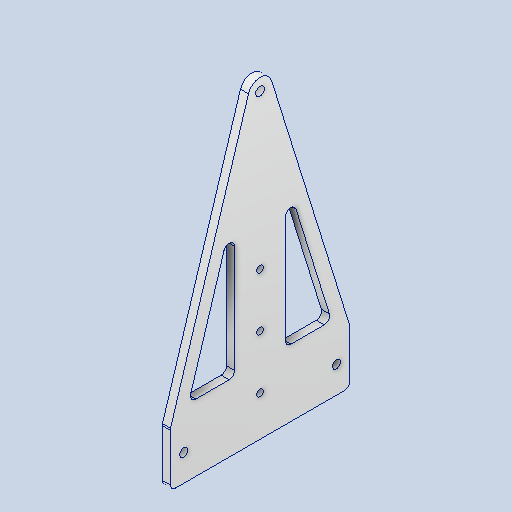
# Autodesk Inventor part: odom_v1_Plate_5
Saved by Autodesk Inventor 2025.2 (Build 292293000, 293)
## iProperties
Created: 2025-04-01
Part Number: odom_v1_Plate_5
Material: アルミニウム 6061
Document SubType Name: Modeling
Designer: haruy
Density: 2.7 g/cm^3
Appearance: アルミニウム - フラット
Author: haruy
Autodesk Inventor part; units mm, degrees
ref_plane "YZ Plane" through (0, 0, 0) normal (1, 0, 0) x (0, 1, 0)
ref_plane "XZ Plane" through (0, 0, 0) normal (0, 1, 0) x (-1, 0, 0)
ref_plane "XY Plane" through (0, 0, 0) normal (0, 0, 1) x (1, 0, 0)
derived "odom_v1_Sketch_Base.ipt"
sketch "スケッチ1" plane through (300, 0, 0) normal (1, 0, 0) x (0, 1, 0)
  line L0 (0, 0) -> (20, 0)
  line L1 (20, 0) -> (20, -192.6893)
  line L2 (20, -192.6893) -> (0, -192.6893)
  line L3 (0, -192.6893) -> (0, 0)
  line L4 (-77, 0) -> (-77, -265.1297)
  circle A0 centre (7.5, -57.9764) radius 1.6
  circle A1 centre (7.5, -93.4764) radius 1.6
  line L5 (-20, -52.2264) -> (-66, -52.2264)
  line L6 (-66, -52.2264) -> (-66, -57.2264)
  line L7 (-66, -57.2264) -> (-20, -57.2264)
  line L8 (-20, -57.2264) -> (-20, -52.2264)
  line L9 (-20, -94.2264) -> (-66, -94.2264)
  line L10 (-66, -94.2264) -> (-66, -99.2264)
  line L11 (-66, -99.2264) -> (-20, -99.2264)
  line L12 (-20, -99.2264) -> (-20, -94.2264)
  line L13 (-19.371, -66.7264) -> (-77, -66.7264)
  line L14 (-77, -66.7264) -> (-77, -84.7264)
  line L15 (-77, -84.7264) -> (-19.371, -84.7264)
  line L16 (-19.371, -84.7264) -> (-19.371, -66.7264)
  line L17 (-41.1855, -57.2264) -> (-55.1855, -57.2264)
  line L18 (-55.1855, -57.2264) -> (-55.1855, -58.0264)
  line L19 (-55.1855, -58.0264) -> (-41.1855, -58.0264)
  line L20 (-41.1855, -58.0264) -> (-41.1855, -57.2264)
  line L21 (-48.1855, -66.7264) -> (-48.1855, -84.7264)
  line L22 (-55.1855, -94.2264) -> (-41.1855, -94.2264)
  line L23 (-41.1855, -94.2264) -> (-41.1855, -93.4264)
  line L24 (-41.1855, -93.4264) -> (-55.1855, -93.4264)
  line L25 (-55.1855, -93.4264) -> (-55.1855, -94.2264)
  circle A2 centre (48, -75.7264) radius 1.65
  circle A3 centre (-17, -75.7264) radius 2
  line L26 (48, -75.7264) -> (-17, -75.7264)
  line L27 (33.5, -67.2264) -> (-12, -67.2264)
  line L28 (-12, -67.2264) -> (-12, -84.2264)
  line L29 (-12, -84.2264) -> (33.5, -84.2264)
  line L30 (33.5, -84.2264) -> (33.5, -67.2264)
  line L31 (-12, -73.7264) -> (-20, -73.7264)
  line L32 (-20, -73.7264) -> (-20, -77.7264)
  line L33 (-20, -77.7264) -> (-12, -77.7264)
  line L34 (-12, -77.7264) -> (-12, -73.7264)
  line L35 (-2, -71.2264) -> (-57, -71.2264)
  line L36 (-57, -71.2264) -> (-57, -80.2264)
  line L37 (-57, -80.2264) -> (-2, -80.2264)
  line L38 (-2, -80.2264) -> (-2, -71.2264)
  circle A4 centre (-9.5, -75.7264) radius 1.25
  circle A5 centre (-29.5, -75.7264) radius 1.25
  circle A6 centre (-49.5, -75.7264) radius 1.25
  line L39 (-52, -65.7264) -> (-22, -65.7264)
  line L40 (-22, -65.7264) -> (-22, -85.7264)
  line L41 (-22, -85.7264) -> (-52, -85.7264)
  line L42 (-52, -85.7264) -> (-52, -65.7264)
  line L43 (-43, -52.2264) -> (-43, -57.2264)
  circle A7 centre (-33, -54.7264) radius 1.5
  line L44 (-29.5, -75.7264) -> (-49.5, -75.7264)
  circle A8 centre (-53, -54.7264) radius 1.5
  circle A9 centre (-53, -96.7264) radius 1.5
  circle A10 centre (-33, -96.7264) radius 1.5
  line L45 (-44.5, -42.2264) -> (-64.5, -42.2264)
  line L46 (-64.5, -42.2264) -> (-64.5, -109.2264)
  line L47 (-64.5, -109.2264) -> (-44.5, -109.2264)
  line L48 (-44.5, -109.2264) -> (-44.5, -42.2264)
  circle A11 centre (-54.5, -47.2264) radius 1.5
  circle A12 centre (-54.5, -104.2264) radius 1.5
  circle A13 centre (48, -75.7264) radius 4.5
  line L49 (48, -71.2264) -> (-2, -71.2264)
  line L50 (-2, -80.2264) -> (48, -80.2264)
  line L51 (-44.5, -42.2264) -> (49.3372, -71.4297)
  line L52 (-39.5, -37.2264) -> (-69.5, -37.2264)
  line L53 (-69.5, -37.2264) -> (-69.5, -114.2264)
  line L54 (-69.5, -114.2264) -> (-39.5, -114.2264)
  line L55 (-39.5, -114.2264) -> (-39.5, -37.2264)
  line L56 (-45.9858, -47.0006) -> (47.8514, -76.2038)
  line L57 (48, -66.2264) -> (-2, -66.2264)
  line L58 (-62, -66.2264) -> (3, -66.2264)
  line L59 (3, -66.2264) -> (3, -85.2264)
  line L60 (3, -85.2264) -> (-62, -85.2264)
  line L61 (-62, -85.2264) -> (-62, -66.2264)
  line L62 (33.5, -84.2264) -> (-12, -84.2264)
  line L63 (-44.5, -109.2264) -> (49.3372, -80.0232)
  line L64 (-39.5, -37.2264) -> (-39.5, -114.2264)
  line L65 (-45.9858, -104.4523) -> (47.8514, -75.249)
  line L66 (48, -85.2264) -> (-2, -85.2264)
  line L67 (-62, -85.2264) -> (3, -85.2264)
  point P0 (-44.5, -71.2264)
  point P1 (-44.5, -80.2264)
  point P2 (-39.5, -85.2264)
  point P3 (15.7916, -85.2264)
  point P4 (-20, -96.3652)
  point P5 (-29.1938, -99.2264)
  point P6 (-39.5, -102.4338)
  point P7 (49.3372, -80.0232)
  point P8 (-39.5, -49.019)
  point P9 (15.7916, -66.2264)
  point P10 (-2, -66.2264)
  point P11 (-39.5, -66.2264)
  point P12 (8.853, -58.8305)
  point P13 (5.9013, -57.9119)
  dimension "d1" = 20
  dimension "d2" = 12.5
  dimension "d3" = 3
  dimension "d4" = 3
  dimension "d5" = 10
  dimension "d7" = 10
  dimension "d10" = 5
  dimension "d11" = 5
  dimension "d12" = 5
  dimension "d13" = 5
  dimension "d14" = 9
  dimension "d17" = 5
  dimension "d18" = 5
  dimension "d19" = 5
  dimension "d20" = 5
  measures "d1" distance of L47.end L46.end
  measures "d2" distance between parallel lines of L4 L46
  measures "d3" diameter of A11
  measures "d4" diameter of A12
  measures "d5" distance from line of A11.centre L46
  measures "d7" distance from line of A12.centre L46
  measures "d10" distance from line of A11.centre L45
  measures "d11" distance from line of L47 A12.centre
  measures "d12" distance from line of L5 A11.centre
  measures "d13" distance from line of A12.centre L11
  measures "d14" diameter of A13
  measures "d17" distance between parallel lines of L48 L55
  measures "d18" distance between parallel lines of L51 L56
  measures "d19" distance between parallel lines of L49 L57
  measures "d20" distance between parallel lines of L35 L58
extrude "押し出し1" add sketch "スケッチ1" against normal blind 3 contours L51 A0 L1 L57 L56 L3 | L3 L56 L8 L5 L55 L51 | L51 L57 L1 | L55 L56 L48 L51 | L51 A0 | L57 L51 A13 L49 L30 L27 L1 | L1 L27 L56 L57 | L57 L59 L27 L3 | L3 L27 L28 L35 L16 L13 L40 L58 L57 | L56 L5 L8 | L56 L27 L59 L57 | L48 L5 L46 L45 | L55 L5 L48 L56 | L27 L30 L49 L56 L1 | L1 L56 L27 | L65 A2 L26 | L26 A2 L56 | A13 L65 L56 | L27 L59 L49 L3 | L3 L49 L35 L28 L27 | L56 L1 L49 L59 L27 | L55 L7 L43 L5 | L56 L49 L1 | A13 L56 L30 L49 | L49 L59 L26 L3 | L3 L26 L38 L49 | L40 L13 L55 L58 | L55 L39 L48 L19 L20 L7 | L5 L48 L7 L46 | L5 L43 L7 L48 | L49 L56 L30 L26 L1 | L1 L26 L59 L49 | L49 L30 L56 | L63 L66 L1 L29 L30 L50 A13 | L56 L26 A13 | A13 L26 L30 L56 | L26 L59 L50 L3 | L3 L50 L38 L26 | L38 L26 A4 L28 L35 | L28 L31 L16 L35 | L40 L35 L55 L13 | L13 L16 L35 L40 | L58 L48 L39 L55 | L55 L13 L48 L58 | L20 L19 L48 L7 | L7 L18 L19 L48 L39 L42 L58 L61 L13 L46 | L48 L19 L18 L7 | L13 L61 L15 L46 | L26 L30 L65 L50 L1 | L1 L50 L59 L26 | L50 L30 L65 A13 | L63 L1 L66 | A13 L65 L30 L26 | L26 L65 A13 | L50 L59 L29 L3 | L3 L29 L28 L37 L50 | L38 L37 L28 L26 A4 | L28 L26 A3 L31 | L16 L31 L32 L33 L37 L40 L35 | L55 L35 L48 L13 | L40 L37 L55 L35 | L58 L42 L39 L48 | L48 L13 L42 L58 | L61 L58 L42 L13 | L13 L42 L35 L36 L37 L15 L61 | L15 L61 L60 L42 L41 L48 L24 L25 L9 L46 | L50 L65 L1 | L1 L65 L29 L59 L50 | L50 L65 L30 | L30 L29 L1 L65 L50 | L63 A1 L3 L65 L66 L1 | L66 L65 L29 L1 | L29 L59 L60 L3 | L3 L60 L40 L15 L16 L37 L28 L29 | L28 L33 A3 L26 | A3 | A3 L33 L16 L31 | L16 L33 L32 L31 | L48 L35 L21 L13 | L55 L44 L48 L35 | L40 L15 L55 L37 | L37 L16 L15 L40 | L13 L21 L35 L42 | L15 L42 L60 L61 | L9 L48 L11 L46 | L1 L29 L65 | L63 A1 | L66 L59 L29 L65 | L37 L16 L33 L28 | L48 L44 L21 L35 | L55 L37 L48 L44 | L55 L15 L48 L37 | L40 L60 L55 L15 | L42 L37 L36 L35 | L35 L21 L37 L42 | L42 L37 L21 L15 | L15 L48 L60 L42 | L25 L24 L48 L9 | L11 L48 L47 L46 | L63 L48 L65 L55 | L55 L65 L11 L12 L3 L63 | L48 L37 L21 L44 | L48 L15 L21 L37 | L55 L60 L48 L15 | L60 L48 L41 L42 | L48 L24 L23 L9 | L9 L55 L11 L48 | L11 L55 L65 L48 | L12 L11 L65 | L55 L41 L48 L60 | L23 L24 L48 L41 L55 L9 | A8 | A9 picked at (6.9346, -58.4648) picked at (7.3575, -92.2361)
fillet "フィレット1" radius 2 10 edges at (298.5, -39.5, -49.019) (298.5, -39.5, -66.2264) (298.5, 15.7916, -66.2264) (298.5, 15.7916, -85.2264) (298.5, -39.5, -85.2264) (298.5, -39.5, -102.4338) (298.5, -44.5, -109.2264) (298.5, -64.5, -109.2264) (298.5, -64.5, -42.2264) (298.5, -44.5, -42.2264)
equation "\"d4\" = d3"
